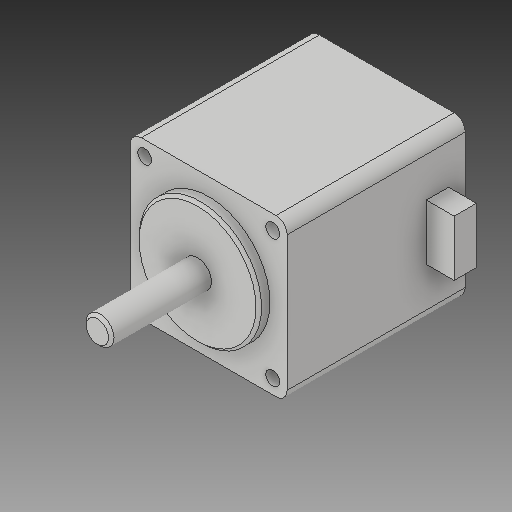
# Autodesk Inventor part: nema11_SY28STH32-0674A
Saved by Autodesk Inventor 2019 (Build 230136000, 136)
## iProperties
Created: 2021-10-13
Part Number: nema11_SY28STH32-0674A
Material: Generic
Document SubType Name: Modeling
Designer: Pokick
Density: 1 g/cm^3
Appearance: Default
Author: Pokick
Autodesk Inventor part; units mm, degrees
ref_plane "YZ Plane" through (0, 0, 0) normal (1, 0, 0) x (0, 1, 0)
ref_plane "XZ Plane" through (0, 0, 0) normal (0, 1, 0) x (-1, 0, 0)
ref_plane "XY Plane" through (0, 0, 0) normal (0, 0, 1) x (1, 0, 0)
sketch "Sketch1" plane through (0, 0, 0) normal (0, 0, 1) x (1, 0, 0)
  line L0 (-14.1, -14.1) -> (14.1, -14.1)
  line L1 (14.1, -14.1) -> (14.1, 14.1)
  line L2 (14.1, 14.1) -> (-14.1, 14.1)
  line L3 (-14.1, 14.1) -> (-14.1, -14.1)
  line L4 (-14.1, -14.1) -> (14.1, 14.1) construction
  line L5 (14.1, -14.1) -> (-14.1, 14.1) construction
  point P0 (0, 0)
  dimension "d0" = 28.2
  dimension "d1" = 28.2
  constraints: 12 end point, 2 midpoint, 2 parallel, 1 horizontal, 1 perpendicular
  measures "d0" distance of L2.end L1.end
  measures "d1" distance of L1.end L0.end
extrude "Extrusion1" add sketch "Sketch1" along normal blind 32
sketch "Sketch2" plane through (0, 0, 32) normal (0, 0, 1) x (1, 0, 0)
  line L0 (-11.5, -11.5) -> (11.5, -11.5) construction
  line L1 (11.5, -11.5) -> (11.5, 11.5) construction
  line L2 (11.5, 11.5) -> (-11.5, 11.5) construction
  line L3 (-11.5, 11.5) -> (-11.5, -11.5) construction
  line L4 (-11.5, -11.5) -> (11.5, 11.5) construction
  line L5 (11.5, -11.5) -> (-11.5, 11.5) construction
  circle A0 centre (-11.5, 11.5) radius 1.25
  line L6 (11.5, -11.5) -> (11.5, 11.5) construction
  line L7 (11.5, 11.5) -> (-11.5, 11.5) construction
  line L8 (-11.5, 11.5) -> (-11.5, -11.5) construction
  line L9 (-11.5, -11.5) -> (11.5, -11.5) construction
  line L10 (11.5, -11.5) -> (-11.5, 11.5) construction
  line L11 (11.5, 11.5) -> (-11.5, -11.5) construction
  circle A1 centre (-11.5, -11.5) radius 1.25
  line L12 (11.5, 11.5) -> (-11.5, 11.5) construction
  line L13 (-11.5, 11.5) -> (-11.5, -11.5) construction
  line L14 (-11.5, -11.5) -> (11.5, -11.5) construction
  line L15 (11.5, -11.5) -> (11.5, 11.5) construction
  line L16 (11.5, 11.5) -> (-11.5, -11.5) construction
  line L17 (-11.5, 11.5) -> (11.5, -11.5) construction
  circle A2 centre (11.5, -11.5) radius 1.25
  line L18 (-11.5, 11.5) -> (-11.5, -11.5) construction
  line L19 (-11.5, -11.5) -> (11.5, -11.5) construction
  line L20 (11.5, -11.5) -> (11.5, 11.5) construction
  line L21 (11.5, 11.5) -> (-11.5, 11.5) construction
  line L22 (-11.5, 11.5) -> (11.5, -11.5) construction
  line L23 (-11.5, -11.5) -> (11.5, 11.5) construction
  circle A3 centre (11.5, 11.5) radius 1.25
  point P0 (0, 0)
  point P1 (0, 0)
  point P2 (0, 0)
  point P3 (0, 0)
  dimension "d4" = 23
  dimension "d5" = 23
  dimension "d6" = 2.5
  dimension "d9" = 360
  constraints: 48 end point, 8 midpoint, 6 coincident, 4 centre point, 2 parallel, 1 horizontal, 1 perpendicular, 51 other
  measures "d4" distance of L2.end L1.end
  measures "d5" distance of L1.end L0.end
  measures "d6" diameter of A0
extrude "Extrusion2" cut sketch "Sketch2" against normal blind 4.5
sketch "Sketch3" plane through (0, 0, 32) normal (0, 0, 1) x (1, 0, 0)
  circle A0 centre (0, 0) radius 11
  dimension "d13" = 22
  constraints: 1 centre point, 1 coincident
  measures "d13" diameter of A0
extrude "Extrusion3" add sketch "Sketch3" along normal blind 2
sketch "Sketch4" plane through (0, 0, 34) normal (0, 0, 1) x (1, 0, 0)
  circle A0 centre (0, 0) radius 2.5
  dimension "d16" = 5
  constraints: 1 centre point, 1 coincident
  measures "d16" diameter of A0
extrude "Extrusion4" add sketch "Sketch4" along normal blind 18
fillet "Fillet1" radius 2 4 edges at (-14.1, 14.1, 16) (14.1, 14.1, 16) (14.1, -14.1, 16) (-14.1, -14.1, 16)
chamfer "Chamfer1" distance 0.5 angle 45 1 edges at (-2.5, 0, 52)
chamfer "Chamfer2" distance 0.5 angle 45 1 edges at (-11, 0, 34)
sketch "Sketch5" plane through (14.1, -12.1, 0) normal (1, 0, 0) x (0, 0, -1)
  line L0 (0, 12.1) -> (-5, 12.1) construction
  line L1 (-7, 7.1) -> (-3, 7.1)
  line L2 (-3, 7.1) -> (-3, 17.1)
  line L3 (-3, 17.1) -> (-7, 17.1)
  line L4 (-7, 17.1) -> (-7, 7.1)
  line L5 (-7, 7.1) -> (-3, 17.1) construction
  line L6 (-3, 7.1) -> (-7, 17.1) construction
  dimension "d26" = 5
  dimension "d27" = 4
  dimension "d28" = 10
  constraints: 14 end point, 2 horizontal, 2 midpoint, 2 parallel, 1 perpendicular
  measures "d26" distance of L0.start L0.end
  measures "d27" distance of L3.end L2.end
  measures "d28" distance of L2.end L1.end
extrude "Extrusion5" add sketch "Sketch5" along normal blind 5
body "Solid1"
